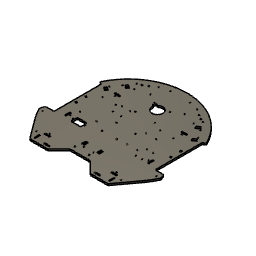
move_base_main_plate (Autodesk Fusion 360 design; units mm, degrees)
Autodesk Fusion 360 part; units mm, degrees
note: some values were not read from the file. Set by a fixed rule: which sketch regions a step uses.
sketch "スケッチ1" plane through (0, 0, 0) normal (0, 1, 0) x (1, 0, 0)
  circle A0 centre (0, 0) radius 220
  dimension "d1" = 440
  constraint coincident A0.centre origin
  measures "d1" diameter of A0
sketch "スケッチ2" plane through (0, 0, 0) normal (0, 1, 0) x (1, 0, 0)
  line L0 (-153.355, -39.3161) -> (-63.355, -39.3161)
  line L1 (-63.355, -39.3161) -> (-63.355, -141.3161)
  line L2 (-63.355, -141.3161) -> (-153.355, -141.3161)
  line L3 (-153.355, -141.3161) -> (-153.355, -39.3161)
  circle A0 centre (0, -150) radius 60.5
  line L4 (-174.2878, 56.0852) -> (-203.2878, 56.0852)
  line L5 (-203.2878, 56.0852) -> (-203.2878, -43.9148)
  line L6 (-203.2878, -43.9148) -> (-174.2878, -43.9148)
  line L7 (-174.2878, -43.9148) -> (-174.2878, 56.0852)
  line L8 (-147.9328, 18.2444) -> (-59.029, 18.2444)
  line L9 (-59.029, 18.2444) -> (-59.029, -18.7556)
  line L10 (-59.029, -18.7556) -> (-147.9328, -18.7556)
  line L11 (-147.9328, -18.7556) -> (-147.9328, 18.2444)
  dimension "d2" = 102
  dimension "d3" = 90
  dimension "d4" = 121
  dimension "d5" = 100
  dimension "d6" = 29
  dimension "d7" = 37
  dimension "d8" = 150
  constraint horizontal L0
  constraint vertical L1
  constraint horizontal L2
  constraint vertical L3
  constraint horizontal L4
  constraint vertical L5
  constraint horizontal L6
  constraint vertical L7
  constraint horizontal L8
  constraint vertical L9
  constraint horizontal L10
  constraint vertical L11
  measures "d2" distance of L0.start L2.end
  measures "d3" distance of L0.start L0.end
  measures "d4" diameter of A0
  measures "d5" distance of L4.end L5.end
  measures "d6" distance of L4.start L4.end
  measures "d7" distance of L8.end L9.end
  measures "d8" distance of A0.centre origin
sketch "スケッチ3" plane through (0, 0, 0) normal (0, 1, 0) x (1, 0, 0)
  line L0 (-159, 75) -> (-159, -75)
  line L1 (-159, -75) -> (-196.1505, -75)
  line L2 (-159, 75) -> (-168.0208, 75)
  line L3 (168.0208, 75) -> (159, 75)
  line L4 (159, 75) -> (159, -75)
  line L5 (159, -75) -> (196.1505, -75)
  arc A0 (168.0208, 75) -> (-168.0208, 75) centre (0, 0) ccw
  arc A1 (-196.1505, -75) -> (196.1505, -75) centre (0, 0) ccw
  circle A2 centre (0, -230) radius 75
  circle A3 centre (0, -210) radius 85
  line L6 (168.7454, -125) -> (68.3017, -260.5952)
  line L7 (-168.7454, -125) -> (-68.3017, -260.5952)
  line L8 (-122.8182, -187) -> (122.8182, -187)
  line L9 (-67, -187) -> (-32, -152)
  line L10 (-32, -152) -> (32, -152)
  line L11 (32, -152) -> (67, -187)
  point P0 (-159, 0)
  point P1 (159, 0)
  point P2 (0, -152)
  dimension "d9" = 150
  dimension "d10" = 159
  dimension "d12" = 159
  dimension "d13" = 184
  dimension "d14" = 210
  dimension "d64" = 150
  dimension "d65" = 230
  dimension "d66" = 210
  dimension "d67" = 170
  dimension "d109" = 187
  dimension "d164" = 64
  dimension "d165" = 35
  dimension "d166" = 135
  dimension "d167" = 135
  constraint vertical L0
  constraint perpendicular L0 L1
  constraint perpendicular L0 L2
  constraint horizontal L3
  constraint perpendicular L3 L4
  constraint perpendicular L4 L5
  constraint midpoint L0 P0
  constraint midpoint L4 P1
  constraint horizontal P1 A0.centre
  constraint horizontal P0 A0.centre
  constraint equal L0 L4
  constraint coincident A0.centre A1.centre
  constraint coincident L3.start A0.start
  constraint coincident L1.end A1.start
  constraint vertical A0.centre A2.centre
  constraint vertical A0.centre A3.centre
  constraint coincident A1 L7.start
  constraint coincident A3 L7.end
  constraint coincident A3 L6.end
  constraint coincident A1 L6.start
  constraint tangent A1 L6
  constraint tangent A3 L6
  constraint tangent A1 L7
  constraint tangent A3 L7
  constraint horizontal L8
  constraint coincident L6 L8.end
  constraint coincident L7 L8.start
  constraint coincident L8 L9.start
  constraint parallel L8 L10
  constraint coincident L8 L11.end
  constraint midpoint L10 P2
  constraint vertical A0.centre P2
  measures "d9" distance of L0.start L0.end
  measures "d10" distance of P0 A0.centre
  measures "d12" distance of P1 A0.centre
  measures "d13" radius of A0
  measures "d14" radius of A1
  measures "d64" diameter of A2
  measures "d65" distance of A0.centre A2.centre
  measures "d66" distance of A0.centre A3.centre
  measures "d67" diameter of A3
  measures "d109" distance of A0.centre L8
  measures "d164" distance of L9.end L10.end
  measures "d165" distance of L8 L10
  measures "d166" angle of L10 L11
  measures "d167" angle of L9 L10
extrude "押し出し1" add sketch "スケッチ3" along normal blind 5 contours L0 L1 L2 L3 L4 L5 A0 A1 A3 L8 | A1 L7 L8 | A3 L8 L9 L10 L11 | A1 L6 L8
sketch "スケッチ8" plane through (0, 5, 0) normal (0, 1, 0) x (-1, 0, 0)
  line L0 (-122.8182, 187) -> (-168.7454, 125)
  arc A0 (-168.7454, 125) -> (-196.1505, 75) centre (0, 0) ccw
  line L1 (-196.1505, 75) -> (-159, 75)
  line L2 (-159, 75) -> (-159, -75)
  arc A1 (-168.0208, -75) -> (168.0208, -75) centre (0, 0) ccw
  line L3 (159, -75) -> (159, 75)
  line L4 (159, 75) -> (196.1505, 75)
  line L5 (168.7454, 125) -> (122.8182, 187)
  line L6 (122.8182, 187) -> (67, 187)
  line L7 (31, -163) -> (-31, -163)
  line L8 (25, -106) -> (-25, -106)
  line L9 (-159, -75) -> (-168.0208, -75)
  line L10 (168.0208, -75) -> (159, -75)
  circle A2 centre (0, 0) radius 165
  line L11 (104.1506, -130.3942) -> (60.8494, -155.3942)
  line L12 (60.8494, -155.3942) -> (49.8494, -136.3416)
  line L13 (49.8494, -136.3416) -> (93.1506, -111.3416)
  line L14 (93.1506, -111.3416) -> (104.1506, -130.3942)
  line L15 (-60.8494, -155.3942) -> (-104.1506, -130.3942)
  line L16 (-104.1506, -130.3942) -> (-93.1507, -111.3416)
  line L17 (-93.1507, -111.3416) -> (-49.8494, -136.3416)
  line L18 (-49.8494, -136.3416) -> (-60.8494, -155.3942)
  line L19 (82.5, -142.8942) -> (0, 0)
  line L20 (0, 0) -> (-82.5, -142.8942)
  line L21 (0, 0) -> (0, -165)
  circle A3 centre (0, -91) radius 17.5
  line L22 (17.0919, -94.7574) -> (12.2438, -103.5036)
  line L23 (12.2438, -103.5036) -> (18.3661, -106.8973)
  line L24 (18.3661, -106.8973) -> (23.2142, -98.1511)
  line L25 (23.2142, -98.1511) -> (17.0919, -94.7574)
  line L26 (0, -91) -> (14.6678, -99.1305)
  line L27 (31, 138) -> (-15, 138)
  line L28 (-15, 138) -> (-15, 52)
  line L29 (-15, 52) -> (31, 52)
  line L30 (31, 52) -> (31, 138)
  line L31 (-30, -52) -> (30, -52)
  line L32 (30, -52) -> (30, 8)
  line L33 (30, 8) -> (-30, 8)
  line L34 (-30, 8) -> (-30, -52)
  line L35 (-30, -52) -> (30, 8) construction
  line L36 (30, -52) -> (-30, 8) construction
  line L37 (-60, -40) -> (-102, -40)
  line L38 (122, -40) -> (80, -40)
  line L39 (-45, -10) -> (-77, -10)
  line L40 (-77, -10) -> (-77, 49.5)
  line L41 (-77, 49.5) -> (-45, 49.5)
  line L42 (-45, 49.5) -> (-45, -10)
  line L43 (92.7583, -134.6621) -> (78.9019, -142.6621)
  line L44 (-78.9019, -142.6621) -> (-92.7583, -134.6621)
  arc A4 (-102.846, 122.5671) -> (102.846, 122.5671) centre (0, 0) ccw
  line L45 (0, 0) -> (102.846, 122.5671)
  line L46 (0, 0) -> (-102.846, 122.5671)
  line L47 (0, 0) -> (131.0643, -91.7722)
  line L48 (139.668, -79.4849) -> (122.4607, -104.0595)
  line L49 (0, 0) -> (-131.0643, -91.7722)
  line L50 (-122.4607, -104.0595) -> (-139.668, -79.4849)
  line L51 (114.185, -114.1349) -> (104.3552, -107.252)
  line L52 (104.3552, -107.252) -> (108.9438, -100.6988)
  line L53 (108.9438, -100.6988) -> (118.7736, -107.5817)
  line L54 (118.7736, -107.5817) -> (114.185, -114.1349)
  line L55 (146.3053, -68.2624) -> (136.4755, -61.3795)
  line L56 (136.4755, -61.3795) -> (131.8869, -67.9327)
  line L57 (131.8869, -67.9327) -> (141.7167, -74.8156)
  line L58 (141.7167, -74.8156) -> (146.3053, -68.2624)
  line L59 (141.7167, -74.8156) -> (118.7736, -107.5817)
  line L60 (-118.7736, -107.5817) -> (-141.7167, -74.8156)
  line L61 (-118.7736, -107.5817) -> (-114.185, -114.1349)
  line L62 (-114.185, -114.1349) -> (-104.3552, -107.252)
  line L63 (-104.3552, -107.252) -> (-108.9438, -100.6988)
  line L64 (-108.9438, -100.6988) -> (-118.7736, -107.5817)
  line L65 (-141.7167, -74.8156) -> (-146.3053, -68.2624)
  line L66 (-146.3053, -68.2624) -> (-136.4755, -61.3795)
  line L67 (-136.4755, -61.3795) -> (-131.8869, -67.9327)
  line L68 (-131.8869, -67.9327) -> (-141.7167, -74.8156)
  line L69 (-90, 32) -> (-110, 32)
  line L70 (-110, 32) -> (-110, 67)
  line L71 (-110, 67) -> (-90, 67)
  line L72 (-90, 67) -> (-90, 32)
  arc A5 (196.1505, 75) -> (168.7454, 125) centre (0, 0) ccw
  line L73 (66, -45.5) -> (40, -45.5)
  line L74 (40, -45.5) -> (40, -17)
  line L75 (40, -17) -> (66, -17)
  line L76 (66, -17) -> (66, -45.5)
  line L77 (67, 187) -> (32, 152)
  line L78 (32, 152) -> (-32, 152)
  line L79 (-32, 152) -> (-67, 187)
  line L80 (-67, 187) -> (-122.8182, 187)
  line L81 (49.8494, -136.3416) -> (58.5096, -131.3416)
  line L82 (58.5096, -131.3416) -> (53.5096, -122.6814)
  line L83 (53.5096, -122.6814) -> (44.8494, -127.6814)
  line L84 (44.8494, -127.6814) -> (49.8494, -136.3416)
  line L85 (-49.8494, -136.3416) -> (-58.5096, -131.3416)
  line L86 (-58.5096, -131.3416) -> (-53.5096, -122.6814)
  line L87 (-53.5096, -122.6814) -> (-44.8494, -127.6814)
  line L88 (-44.8494, -127.6814) -> (-49.8494, -136.3416)
  line L89 (15, 125) -> (-15, 125)
  line L90 (20, 119) -> (-20, 119)
  line L91 (20, 119) -> (28, 119)
  line L92 (28, 119) -> (28, 107)
  line L93 (28, 107) -> (20, 107)
  line L94 (20, 107) -> (20, 119)
  line L95 (-20, 119) -> (-28, 119)
  line L96 (-28, 119) -> (-28, 107)
  line L97 (-28, 107) -> (-20, 107)
  line L98 (-20, 107) -> (-20, 119)
  circle A6 centre (87, 177) radius 1.6
  circle A7 centre (72, 177) radius 1.6
  line L99 (87, 178.6) -> (72, 178.6)
  line L100 (72, 178.6) -> (72, 175.4)
  line L101 (72, 175.4) -> (87, 175.4)
  line L102 (87, 175.4) -> (87, 178.6)
  line L103 (115.4, 177) -> (118.6, 177)
  line L104 (118.6, 177) -> (118.6, 162)
  line L105 (118.6, 162) -> (115.4, 162)
  line L106 (115.4, 162) -> (115.4, 177)
  circle A8 centre (117, 177) radius 1.6
  circle A9 centre (117, 162) radius 1.6
  circle A10 centre (-72, 177) radius 1.6
  circle A11 centre (-87, 177) radius 1.6
  circle A12 centre (-117, 177) radius 1.6
  circle A13 centre (-117, 162) radius 1.6
  line L107 (-72, 175.4) -> (-87, 175.4)
  line L108 (-87, 175.4) -> (-87, 178.6)
  line L109 (-87, 178.6) -> (-72, 178.6)
  line L110 (-72, 178.6) -> (-72, 175.4)
  line L111 (-115.4, 177) -> (-118.6, 177)
  line L112 (-118.6, 177) -> (-118.6, 162)
  line L113 (-118.6, 162) -> (-115.4, 162)
  line L114 (-115.4, 162) -> (-115.4, 177)
  line L115 (75, 75) -> (106, 75)
  line L116 (106, 75) -> (106, 55)
  line L117 (106, 55) -> (75, 55)
  line L118 (75, 55) -> (75, 75)
  line L119 (75, 75) -> (106, 55) construction
  line L120 (106, 75) -> (75, 55) construction
  line L121 (109, 65) -> (72, 65)
  line L122 (117, 35) -> (65, 35)
  point P0 (0, -163)
  point P1 (0, -106)
  point P2 (0, -165)
  point P3 (82.5, -142.8942)
  point P4 (-82.5, -142.8942)
  point P5 (8, 52)
  point P6 (0, -22)
  point P7 (0, -160)
  point P8 (102.846, 122.5671)
  point P9 (-102.846, 122.5671)
  point P10 (131.0643, -91.7722)
  point P11 (-131.0643, -91.7722)
  point P12 (0, -157)
  point P13 (130.2452, -91.1987)
  point P14 (-130.2452, -91.1987)
  point P15 (98.9893, 117.9708)
  point P16 (-98.9893, 117.9708)
  point P17 (0, 125)
  point P18 (0, 119)
  point P19 (90.5, 65)
  dimension "d68" = 163
  dimension "d69" = 62
  dimension "d70" = 50
  dimension "d71" = 57
  dimension "d75" = 330
  dimension "d78" = 30
  dimension "d79" = 30
  dimension "d80" = 50
  dimension "d81" = 35
  dimension "d82" = 15
  dimension "d83" = 7
  dimension "d84" = 10
  dimension "d85" = 61
  dimension "d101" = 22
  dimension "d102" = 86
  dimension "d103" = 46
  dimension "d104" = 52
  dimension "d105" = 8
  dimension "d110" = 60
  dimension "d111" = 22
  dimension "d112" = 42
  dimension "d113" = 60
  dimension "d114" = 80
  dimension "d115" = 40
  dimension "d116" = 32
  dimension "d117" = 59.5
  dimension "d118" = 45
  dimension "d119" = 10
  dimension "d120" = 2
  dimension "d121" = 13
  dimension "d122" = 3
  dimension "d123" = 3
  dimension "d124" = 13
  dimension "d125" = 2
  dimension "d129" = 160
  dimension "d130" = 55
  dimension "d131" = 85
  dimension "d132" = 55
  dimension "d133" = 85
  dimension "d141" = 1
  dimension "d142" = 1
  dimension "d145" = 20
  dimension "d146" = 35
  dimension "d157" = 26
  dimension "d158" = 28.5
  dimension "d159" = 40
  dimension "d160" = 17
  dimension "d175" = 10
  dimension "d176" = 12
  dimension "d178" = 20
  dimension "d179" = 125
  dimension "d180" = 40
  dimension "d181" = 30
  dimension "d182" = 6
  dimension "d183" = 12
  dimension "d184" = 8
  dimension "d185" = 3.2
  dimension "d186" = 3.2
  dimension "d187" = 10
  dimension "d188" = 15
  dimension "d189" = 5
  dimension "d190" = 10
  dimension "d191" = 50
  dimension "d192" = 15
  dimension "d193" = 3.2
  dimension "d194" = 3.2
  dimension "d195" = 5
  dimension "d196" = 10
  dimension "d197" = 15
  dimension "d198" = 50
  dimension "d199" = 10
  dimension "d200" = 15
  dimension "d201" = 31
  dimension "d202" = 20
  dimension "d203" = 37
  dimension "d204" = 75
  dimension "d205" = 65
  dimension "d219" = 8
  dimension "d223" = 90
  dimension "d224" = 32
  dimension "d225" = 52
  dimension "d226" = 65
  dimension "d227" = 35
  constraint horizontal L7
  constraint horizontal L8
  constraint midpoint L7 P0
  constraint midpoint L8 P1
  constraint vertical A0.centre P1
  constraint vertical A0.centre P0
  constraint concentric A0 A2
  constraint coincident A2 P2
  constraint perpendicular L11 L12
  constraint parallel L11 L13
  constraint parallel L12 L14
  constraint perpendicular L15 L16
  constraint parallel L15 L17
  constraint parallel L16 L18
  constraint coincident A2 P3
  constraint coincident A0.centre A1.centre
  constraint coincident A2 P4
  constraint coincident P2 L21.end
  constraint midpoint L11 P3
  constraint midpoint L15 P4
  constraint coincident P4 L20.end
  constraint coincident P3 L19.start
  constraint tangent A2 L11
  constraint tangent A2 L15
  constraint equal L13 L17
  constraint perpendicular L22 L23
  constraint parallel L22 L24
  constraint parallel L23 L25
  constraint coincident A3 L22.end
  constraint coincident A3 L22.start
  constraint vertical P1 A3.centre
  constraint coincident A3.centre L26.start
  constraint perpendicular L22 L26
  constraint coincident L22 L26.end
  constraint vertical L21
  constraint equal L12 L18
  constraint horizontal L27
  constraint vertical L28
  constraint horizontal L29
  constraint midpoint L29 P5
  constraint horizontal L31
  constraint perpendicular L31 L32
  constraint parallel L31 L33
  constraint parallel L32 L34
  constraint coincident L35 P6
  constraint coincident L36 P6
  constraint vertical A0.centre P6
  constraint equal L31 L32
  constraint horizontal L37
  constraint horizontal L38
  constraint equal L37 L38
  constraint collinear L37 L38
  constraint horizontal L39
  constraint vertical L40
  constraint horizontal L41
  constraint vertical L42
  constraint parallel L11 L43
  constraint perpendicular L20 L44
  constraint coincident L21 P7
  constraint coincident P7 A4
  constraint coincident P9 A4.start
  constraint coincident P8 A4.end
  constraint coincident A4 P10
  constraint perpendicular L47 L48
  constraint midpoint L48 P10
  constraint coincident P10 L47.end
  constraint coincident A4 P11
  constraint midpoint L50 P11
  constraint coincident P11 L49.end
  constraint perpendicular L49 L50
  constraint coincident L21 P12
  constraint perpendicular L51 L52
  constraint parallel L51 L53
  constraint parallel L52 L54
  constraint perpendicular L55 L56
  constraint parallel L55 L57
  constraint parallel L56 L58
  constraint coincident L47 P13
  constraint equal L52 L56
  constraint equal L53 L57
  constraint perpendicular L53 L59
  constraint midpoint P13 L59
  constraint perpendicular L47 L59
  constraint perpendicular L57 L59
  constraint midpoint L60 P14
  constraint coincident L49 P14
  constraint perpendicular L49 L60
  constraint perpendicular L61 L62
  constraint parallel L61 L63
  constraint parallel L62 L64
  constraint parallel L60 L61
  constraint perpendicular L65 L66
  constraint parallel L65 L67
  constraint parallel L66 L68
  constraint perpendicular L49 L65
  constraint equal L62 L66
  constraint equal L63 L67
  constraint coincident L46 P16
  constraint coincident L45 P15
  constraint horizontal L69
  constraint vertical L70
  constraint horizontal L71
  constraint vertical L72
  constraint horizontal L73
  constraint vertical L74
  constraint horizontal L75
  constraint vertical L76
  constraint perpendicular L81 L82
  constraint parallel L81 L83
  constraint parallel L82 L84
  constraint coincident L13 L81.end
  constraint perpendicular L85 L86
  constraint parallel L85 L87
  constraint parallel L86 L88
  constraint coincident L17 L85.end
  constraint equal L83 L84
  constraint equal L87 L88
  constraint equal L84 L88
  constraint equal L51 L62
  constraint equal L52 L63
  constraint equal L59 L60
  constraint horizontal L89
  constraint midpoint L89 P17
  constraint vertical A0.centre P17
  constraint horizontal L90
  constraint midpoint L90 P18
  constraint vertical P17 P18
  constraint horizontal L91
  constraint vertical L92
  constraint horizontal L93
  constraint vertical L94
  constraint horizontal L95
  constraint vertical L96
  constraint horizontal L97
  constraint vertical L98
  constraint collinear L93 L97
  constraint equal L93 L97
  constraint horizontal L99
  constraint vertical L100
  constraint horizontal L101
  constraint vertical L102
  constraint horizontal L103
  constraint vertical L104
  constraint horizontal L105
  constraint vertical L106
  constraint tangent A6 L101
  constraint tangent A6 L99
  constraint tangent A7 L99
  constraint tangent A7 L101
  constraint midpoint A6.centre L102
  constraint midpoint A7.centre L100
  constraint tangent L106 A9
  constraint tangent L104 A9
  constraint tangent L104 A8
  constraint tangent L106 A8
  constraint midpoint L105 A9.centre
  constraint midpoint L103 A8.centre
  constraint horizontal L107
  constraint vertical L108
  constraint horizontal L109
  constraint vertical L110
  constraint horizontal L111
  constraint vertical L112
  constraint horizontal L113
  constraint vertical L114
  constraint tangent A10 L107
  constraint tangent A11 L107
  constraint tangent A11 L109
  constraint tangent A10 L109
  constraint tangent A12 L114
  constraint tangent A12 L112
  constraint tangent A13 L112
  constraint tangent A13 L114
  constraint midpoint A13.centre L113
  constraint midpoint A12.centre L111
  constraint midpoint A11.centre L108
  constraint midpoint A10.centre L110
  constraint horizontal L115
  constraint perpendicular L115 L116
  constraint parallel L115 L117
  constraint parallel L116 L118
  constraint coincident L119 P19
  constraint coincident L120 P19
  constraint horizontal L121
  constraint midpoint P19 L121
  constraint vertical L30
  constraint horizontal L122
  measures "d68" distance of A0.centre P0
  measures "d69" distance of L7.start L7.end
  measures "d70" distance of L8.start L8.end
  measures "d71" distance of L7 L8
  measures "d75" diameter of A2
  measures "d78" angle of L19 L21
  measures "d79" angle of L20 L21
  measures "d80" distance of L12.end L13.end
  measures "d81" diameter of A3
  measures "d82" distance of L8 A3.centre
  measures "d83" distance of L22.start L24.end
  measures "d84" distance of L23.end L24.end
  measures "d85" angle of L21 L26
  measures "d101" distance of L11.start L13.end
  measures "d102" distance of L27.end L28.end
  measures "d103" distance of L28.end L29.end
  measures "d104" distance of A0.centre L29
  measures "d105" horizontal distance of A0.centre P5
  measures "d110" distance of L31.end L32.end
  measures "d111" distance of A0.centre P6
  measures "d112" distance of L37.start L37.end
  measures "d113" horizontal distance of A0.centre L37.start
  measures "d114" horizontal distance of A0.centre L38.end
  measures "d115" distance of A0.centre L37
  measures "d116" distance of L39.start L39.end
  measures "d117" distance of L39.end L40.end
  measures "d118" distance of A0.centre L42
  measures "d119" distance of A0.centre L39
  measures "d120" distance of L11 L43
  measures "d121" distance of L19 L43.start
  measures "d122" distance of L19 L43.end
  measures "d123" distance of L20 L44.start
  measures "d124" distance of L20 L44.end
  measures "d125" distance of L15 L44
  measures "d129" radius of A4
  measures "d130" angle of L21 L47
  measures "d131" angle of L45 L47
  measures "d132" angle of L21 L49
  measures "d133" angle of L46 L49
  measures "d141" distance of L48 L59
  measures "d142" distance of L50 L60
  measures "d145" distance of L69.start L69.end
  measures "d146" distance of L69.start L71.end
  measures "d157" distance of L73.start L73.end
  measures "d158" distance of L73.start L75.end
  measures "d159" distance of A0.centre L74
  measures "d160" distance of A0.centre L75
  measures "d175" distance of L12.end L83.end
  measures "d176" distance of L55.start L55.end
  measures "d178" distance of L47 L57
  measures "d179" distance of A0.centre L89
  measures "d180" distance of L90.start L90.end
  measures "d181" distance of L89.start L89.end
  measures "d182" distance of L89 L90
  measures "d183" distance of L91.end L92.end
  measures "d184" distance of L92.end L93.end
  measures "d185" diameter of A6
  measures "d186" diameter of A8
  measures "d187" distance of L6 A6.centre
  measures "d188" distance of A6.centre A7.centre
  measures "d189" horizontal distance of L6.end A7.centre
  measures "d190" vertical distance of L6.end A8.centre
  measures "d191" horizontal distance of L6.end A8.centre
  measures "d192" distance of A8.centre A9.centre
  measures "d193" diameter of A10
  measures "d194" diameter of A13
  measures "d195" horizontal distance of L79.end A10.centre
  measures "d196" vertical distance of L79.end A10.centre
  measures "d197" distance of A10.centre A11.centre
  measures "d198" horizontal distance of L79.end A12.centre
  measures "d199" vertical distance of L79.end A12.centre
  measures "d200" distance of A12.centre A13.centre
  measures "d201" distance of L116.end L117.end
  measures "d202" distance of L115.end L116.end
  measures "d203" distance of L121.start L121.end
  measures "d204" distance of A0.centre L118
  measures "d205" distance of A0.centre L121
  measures "d219" distance of L62.end L63.end
  measures "d223" distance of A0.centre L72
  measures "d224" distance of A0.centre L69
  measures "d225" distance of L122.start L122.end
  measures "d226" horizontal distance of A0.centre L122.end
  measures "d227" distance of A0.centre L122
hole "穴5" at (25, 5, -106) at (-25, 5, -106) at (-31, 5, -163) at (31, 5, -163) at (-104.1506, 5, -130.3942) at (-93.1506, 5, -111.3416) at (-60.8494, 5, -155.3942) at (60.8494, 5, -155.3942) at (104.1506, 5, -130.3942) at (93.1507, 5, -111.3416) at (60, 5, -40) at (102, 5, -40) at (-80, 5, -40) at (-122, 5, -40) at (45, 5, -10) at (77, 5, -10) at (77, 5, 49.5) at (45, 5, 49.5) at (-122.4607, 5, -104.0595) at (-139.668, 5, -79.4849) at (122.4607, 5, -104.0595) at (139.668, 5, -79.4849) at (90, 5, 32) at (110, 5, 32) at (110, 5, 67) at (90, 5, 67) at (-30, 5, -52) at (-30, 5, 8) at (30, 5, 8) at (30, 5, -52) at (-66, 5, -45.5) at (-40, 5, -45.5) at (-40, 5, -17) at (-66, 5, -17) at (-53.5096, 5, -122.6814) at (53.5096, 5, -122.6814) at (-15, 5, 125) at (15, 5, 125) direction (0, -1, 0) diameter 3.2 end through all
extrude "押し出し2" cut sketch "スケッチ8" against normal through all contours A4 L66 L67 L68 | A4 L65 L66 L68 | A4 L55 L57 L58 | A4 L55 L56 L57 | A4 L61 L62 L64 | A4 L62 L63 L64 | A4 L51 L52 L53 | A4 L51 L53 L54 | L21 A3 L22 L26 | L8 L21 A3 | L8 L21 A3 L22 L26 | L8 L21 A3 | L8 L21 A3 | A3 L22 | L8 A3 L23 L24 L25 | L8 L23 L24 | L91 L92 L93 L94 | L95 L96 L97 L98 | A6 L102 | A6 L102 | A6 A7 L99 L101 | A7 L100 | A7 L100 | L103 A8 | L104 L106 A8 A9 | L103 A8 | L105 A9 | L105 A9 | A10 L110 | A10 L110 | A10 A11 L107 L109 | A11 L108 | A11 L108 | A12 L111 | A12 A13 L112 L114 | A12 L111 | A13 L113 | A13 L113 | L115 L116 L118 L121 | L116 L117 L118 L121
sketch "スケッチ9" plane through (0, 5, 0) normal (0, 1, 0) x (-1, 0, 0)
  line L0 (23.2142, -98.1511) -> (18.3661, -106.8973)
  line L1 (18.3661, -106.8973) -> (12.2438, -103.5036)
  arc A0 (17.0919, -94.7574) -> (12.2438, -103.5036) centre (0, -91) ccw
  line L2 (17.0919, -94.7574) -> (23.2142, -98.1511)
  circle A1 centre (-104.1506, -130.3942) radius 1.6
  circle A2 centre (104.1506, -130.3942) radius 1.6
  circle A3 centre (31, -163) radius 1.6
  circle A4 centre (-25, -106) radius 1.6
  circle A5 centre (25, -106) radius 1.6
  circle A6 centre (-31, -163) radius 1.6
  circle A7 centre (93.1506, -111.3416) radius 1.6
  circle A8 centre (60.8494, -155.3942) radius 1.6
  circle A9 centre (-60.8494, -155.3942) radius 1.6
  circle A10 centre (-93.1507, -111.3416) radius 1.6
  line L3 (-122.8182, 187) -> (-168.7454, 125)
  arc A11 (-168.7454, 125) -> (-196.1505, 75) centre (0, 0) ccw
  line L4 (-196.1505, 75) -> (-159, 75)
  line L5 (-159, 75) -> (-159, -75)
  line L6 (-159, -75) -> (-168.0208, -75)
  arc A12 (-168.0208, -75) -> (168.0208, -75) centre (0, 0) ccw
  line L7 (168.0208, -75) -> (159, -75)
  line L8 (159, -75) -> (159, 75)
  line L9 (159, 75) -> (196.1505, 75)
  line L10 (168.7454, 125) -> (122.8182, 187)
  line L11 (122.8182, 187) -> (67, 187)
  line L12 (-130, -70) -> (130, -70)
  line L13 (130, -70) -> (130, 150)
  line L14 (130, 150) -> (-130, 150)
  line L15 (-130, 150) -> (-130, -70)
  line L16 (-130, -70) -> (130, 150) construction
  line L17 (130, -70) -> (-130, 150) construction
  line L18 (123, 60) -> (123, -63)
  line L19 (123, -63) -> (-123, -63)
  line L20 (-123, -63) -> (-123, 60)
  circle A13 centre (80, -40) radius 1.6
  circle A14 centre (-60, -40) radius 1.6
  circle A15 centre (-102, -40) radius 1.6
  circle A16 centre (122, -40) radius 1.6
  circle A17 centre (-77, 49.5) radius 1.6
  circle A18 centre (-45, -10) radius 1.6
  circle A19 centre (-77, -10) radius 1.6
  circle A20 centre (-45, 49.5) radius 1.6
  circle A21 centre (-122.4607, -104.0595) radius 1.6
  circle A22 centre (122.4607, -104.0595) radius 1.6
  circle A23 centre (139.668, -79.4849) radius 1.6
  circle A24 centre (-139.668, -79.4849) radius 1.6
  line L21 (-108.9438, -100.6988) -> (-104.3552, -107.252)
  line L22 (-104.3552, -107.252) -> (-114.185, -114.1349)
  line L23 (-114.185, -114.1349) -> (-118.7736, -107.5817)
  line L24 (-118.7736, -107.5817) -> (-108.9438, -100.6988)
  line L25 (141.7167, -74.8156) -> (131.8869, -67.9327)
  line L26 (131.8869, -67.9327) -> (136.4755, -61.3795)
  line L27 (136.4755, -61.3795) -> (146.3053, -68.2624)
  line L28 (146.3053, -68.2624) -> (141.7167, -74.8156)
  line L29 (118.7736, -107.5817) -> (114.185, -114.1349)
  line L30 (114.185, -114.1349) -> (104.3552, -107.252)
  line L31 (104.3552, -107.252) -> (108.9438, -100.6988)
  line L32 (108.9438, -100.6988) -> (118.7736, -107.5817)
  line L33 (-131.8869, -67.9327) -> (-141.7167, -74.8156)
  line L34 (-141.7167, -74.8156) -> (-146.3053, -68.2624)
  line L35 (-146.3053, -68.2624) -> (-136.4755, -61.3795)
  line L36 (-136.4755, -61.3795) -> (-131.8869, -67.9327)
  circle A25 centre (-110, 67) radius 1.6
  circle A26 centre (-90, 32) radius 1.6
  circle A27 centre (-110, 32) radius 1.6
  circle A28 centre (-90, 67) radius 1.6
  arc A29 (196.1505, 75) -> (168.7454, 125) centre (0, 0) ccw
  circle A30 centre (-30, 8) radius 1.6
  circle A31 centre (30, -52) radius 1.6
  circle A32 centre (30, 8) radius 1.6
  circle A33 centre (-30, -52) radius 1.6
  line L37 (105, 142.5) -> (-105, 142.5)
  circle A34 centre (40, -17) radius 1.6
  circle A35 centre (66, -45.5) radius 1.6
  circle A36 centre (40, -45.5) radius 1.6
  circle A37 centre (66, -17) radius 1.6
  line L38 (97, -72) -> (113, -72)
  line L39 (113, -72) -> (113, -68)
  line L40 (113, -68) -> (97, -68)
  line L41 (97, -68) -> (97, -72)
  line L42 (97, -72) -> (113, -68) construction
  line L43 (113, -72) -> (97, -68) construction
  line L44 (-113, -72) -> (-97, -72)
  line L45 (-97, -72) -> (-97, -68)
  line L46 (-97, -68) -> (-113, -68)
  line L47 (-113, -68) -> (-113, -72)
  line L48 (-113, -72) -> (-97, -68) construction
  line L49 (-97, -72) -> (-113, -68) construction
  line L50 (97, 148) -> (113, 148)
  line L51 (113, 148) -> (113, 152)
  line L52 (113, 152) -> (97, 152)
  line L53 (97, 152) -> (97, 148)
  line L54 (97, 148) -> (113, 152) construction
  line L55 (113, 148) -> (97, 152) construction
  line L56 (-113, 148) -> (-97, 148)
  line L57 (-97, 148) -> (-97, 152)
  line L58 (-97, 152) -> (-113, 152)
  line L59 (-113, 152) -> (-113, 148)
  line L60 (-113, 148) -> (-97, 152) construction
  line L61 (-97, 148) -> (-113, 152) construction
  line L62 (-132, 52) -> (-128, 52)
  line L63 (-128, 52) -> (-128, 68)
  line L64 (-128, 68) -> (-132, 68)
  line L65 (-132, 68) -> (-132, 52)
  line L66 (-132, 52) -> (-128, 68) construction
  line L67 (-128, 52) -> (-132, 68) construction
  line L68 (128, 52) -> (132, 52)
  line L69 (132, 52) -> (132, 68)
  line L70 (132, 68) -> (128, 68)
  line L71 (128, 68) -> (128, 52)
  line L72 (128, 52) -> (132, 68) construction
  line L73 (132, 52) -> (128, 68) construction
  line L74 (67, 187) -> (32, 152)
  line L75 (32, 152) -> (-32, 152)
  line L76 (-32, 152) -> (-67, 187)
  line L77 (-67, 187) -> (-122.8182, 187)
  circle A38 centre (53.5096, -122.6814) radius 1.6
  circle A39 centre (-53.5096, -122.6814) radius 1.6
  circle A40 centre (15, 125) radius 1.6
  circle A41 centre (-15, 125) radius 1.6
  line L78 (20, 107) -> (20, 119)
  line L79 (20, 119) -> (28, 119)
  line L80 (28, 119) -> (28, 107)
  line L81 (28, 107) -> (20, 107)
  line L82 (-20, 107) -> (-28, 107)
  line L83 (-28, 107) -> (-28, 119)
  line L84 (-28, 119) -> (-20, 119)
  line L85 (-20, 119) -> (-20, 107)
  arc A42 (72, 178.6) -> (72, 175.4) centre (72, 177) ccw
  line L86 (72, 178.6) -> (87, 178.6)
  arc A43 (87, 175.4) -> (87, 178.6) centre (87, 177) ccw
  line L87 (87, 175.4) -> (72, 175.4)
  line L88 (118.6, 177) -> (118.6, 162)
  arc A44 (115.4, 162) -> (118.6, 162) centre (117, 162) ccw
  line L89 (115.4, 162) -> (115.4, 177)
  arc A45 (118.6, 177) -> (115.4, 177) centre (117, 177) ccw
  line L90 (-72, 175.4) -> (-87, 175.4)
  arc A46 (-87, 178.6) -> (-87, 175.4) centre (-87, 177) ccw
  line L91 (-87, 178.6) -> (-72, 178.6)
  arc A47 (-72, 175.4) -> (-72, 178.6) centre (-72, 177) ccw
  arc A48 (-118.6, 162) -> (-115.4, 162) centre (-117, 162) ccw
  line L92 (-118.6, 162) -> (-118.6, 177)
  arc A49 (-115.4, 177) -> (-118.6, 177) centre (-117, 177) ccw
  line L93 (-115.4, 177) -> (-115.4, 162)
  line L94 (75, 55) -> (75, 75)
  line L95 (75, 75) -> (106, 75)
  line L96 (106, 75) -> (106, 55)
  line L97 (106, 55) -> (75, 55)
  line L98 (149.05, -15.6) -> (130, -15.6)
  line L99 (130, -15.6) -> (130, 15.6)
  line L100 (130, 15.6) -> (149.05, 15.6)
  line L101 (149.05, 15.6) -> (149.05, -15.6)
  line L102 (-130, -15.6) -> (-149.05, -15.6)
  line L103 (-149.05, -15.6) -> (-149.05, 15.6)
  line L104 (-149.05, 15.6) -> (-130, 15.6)
  line L105 (-130, 15.6) -> (-130, -15.6)
  point P0 (0, 40)
  point P1 (105, -63)
  point P2 (-105, -63)
  point P3 (105, -70)
  point P4 (-105, -70)
  point P5 (105, 150)
  point P6 (-105, 150)
  point P7 (-130, 60)
  point P8 (130, 60)
  point P9 (130, 0)
  point P10 (-130, 0)
  dimension "d89" = 40
  dimension "d90" = 260
  dimension "d91" = 220
  dimension "d92" = 60
  dimension "d93" = 105
  dimension "d94" = 105
  dimension "d95" = 7
  dimension "d96" = 7
  dimension "d97" = 7
  dimension "d156" = 7.5
  dimension "d161" = 16
  dimension "d162" = 4
  dimension "d231" = 19.05
  dimension "d232" = 31.2
  constraint horizontal L12
  constraint perpendicular L12 L13
  constraint parallel L12 L14
  constraint parallel L13 L15
  constraint coincident L16 P0
  constraint coincident L17 P0
  constraint vertical A11.centre P0
  constraint vertical L18
  constraint perpendicular L18 L19
  constraint perpendicular L19 L20
  constraint coincident L19 P1
  constraint coincident L19 P2
  constraint horizontal L18.start L20.end
  constraint horizontal L37
  constraint vertical P1 L37.start
  constraint vertical P2 L37.end
  constraint horizontal L38
  constraint perpendicular L38 L39
  constraint parallel L38 L40
  constraint parallel L39 L41
  constraint coincident L42 P3
  constraint coincident L43 P3
  constraint coincident L12 P3
  constraint vertical P1 P3
  constraint horizontal L44
  constraint perpendicular L44 L45
  constraint parallel L44 L46
  constraint parallel L45 L47
  constraint coincident L48 P4
  constraint coincident L49 P4
  constraint coincident L12 P4
  constraint vertical P2 P4
  constraint horizontal L50
  constraint perpendicular L50 L51
  constraint parallel L50 L52
  constraint parallel L51 L53
  constraint coincident L54 P5
  constraint coincident L55 P5
  constraint coincident L14 P5
  constraint horizontal L56
  constraint perpendicular L56 L57
  constraint parallel L56 L58
  constraint parallel L57 L59
  constraint coincident L60 P6
  constraint coincident L61 P6
  constraint coincident L14 P6
  constraint horizontal L62
  constraint perpendicular L62 L63
  constraint parallel L62 L64
  constraint parallel L63 L65
  constraint coincident L66 P7
  constraint coincident L67 P7
  constraint coincident L15 P7
  constraint horizontal L68
  constraint perpendicular L68 L69
  constraint parallel L68 L70
  constraint parallel L69 L71
  constraint coincident L72 P8
  constraint coincident L73 P8
  constraint coincident L13 P8
  constraint horizontal L18.start P8
  constraint horizontal L20.end P7
  constraint vertical L37.end P6
  constraint vertical L37.start P5
  constraint equal L40 L46
  constraint equal L40 L71
  constraint equal L50 L71
  constraint equal L46 L63
  constraint equal L56 L63
  constraint equal L41 L45
  constraint equal L45 L62
  constraint equal L59 L62
  constraint equal L41 L68
  constraint equal L51 L68
  constraint horizontal L98
  constraint vertical L99
  constraint horizontal L100
  constraint vertical L101
  constraint midpoint L99 P9
  constraint horizontal A11.centre P9
  constraint coincident L13 P9
  constraint horizontal L102
  constraint vertical L103
  constraint horizontal L104
  constraint vertical L105
  constraint midpoint L105 P10
  constraint horizontal A11.centre P10
  constraint coincident L15 P10
  constraint equal L98 L102
  constraint equal L101 L103
  measures "d89" distance of A11.centre P0
  measures "d90" distance of L12.start L12.end
  measures "d91" distance of L12.start L14.end
  measures "d92" vertical distance of A11.centre L18.start
  measures "d93" horizontal distance of A11.centre P1
  measures "d94" horizontal distance of A11.centre P2
  measures "d95" distance of L12 L19
  measures "d96" distance of L15 L20
  measures "d97" distance of L13 L18
  measures "d156" distance of L14 L37
  measures "d161" distance of L38.start L38.end
  measures "d162" distance of L38.start L40.end
  measures "d231" distance of L98.start L98.end
  measures "d232" distance of L98.start L100.end
hole "穴6" at (-123, 5, 60) at (-105, 5, -63) at (105, 5, -63) at (123, 5, 60) at (-105, 5, 142.5) at (105, 5, 142.5) at (-109, 5, 65) at (-72, 5, 65) direction (0, -1, 0) diameter 3.2 end through all
hole "穴7" at (15, 5, 52) at (-31, 5, 52) at (-31, 5, 138) at (15, 5, 138) at (92.7583, 5, -134.6621) at (78.9019, 5, -142.6621) at (-92.7583, 5, -134.6621) at (-78.9019, 5, -142.6621) direction (0, -1, 0) diameter 4.3 end through all
chamfer "面取り1" distance 10 distance2 15 1 edges at (-196.1505, 2.5, 75) measured on face at (-171.3835, 1.6667, 75)
chamfer "面取り2" distance 15 distance2 10 1 edges at (196.1505, 2.5, 75) measured on face at (172.4502, 1.6667, 119.837)
fillet "フィレット1" radius 3 20 edges at (168.0208, 2.5, -75) (159, 2.5, -75) (159, 2.5, 75) (-159, 2.5, 75) (-159, 2.5, -75) (-168.0208, 2.5, -75) (-122.8182, 2.5, 187) (122.8182, 2.5, 187) (190.2963, 2.5, 88.8105) (186.1505, 2.5, 75) (-190.2963, 2.5, 88.8105) (-186.1505, 2.5, 75) (-67, 2.5, 187) (-32, 2.5, 152) (67, 2.5, 187) (32, 2.5, 152) (-75, 2.5, 55) (-106, 2.5, 55) (-106, 2.5, 75) (-75, 2.5, 75)
extrude "押し出し3" cut sketch "スケッチ9" against normal through all contours L12 L45 L46 L47 | L12 L44 L45 L47 | L12 L39 L40 L41 | L12 L38 L39 L41 | L15 L62 L64 L65 | L15 L62 L63 L64 | L14 L57 L58 L59 | L14 L56 L57 L59 | L13 L68 L70 L71 | L13 L68 L69 L70 | L14 L51 L52 L53 | L14 L50 L51 L53
sketch "スケッチ10" plane through (0, 0, 0) normal (0, -1, 0) x (1, 0, 0)
  line L0 (97, 152) -> (113, 152)
  line L1 (113, 152) -> (113, 148)
  line L2 (113, 148) -> (97, 148)
  line L3 (97, 148) -> (97, 152)
  line L4 (-113, -68) -> (-97, -68)
  line L5 (-97, -68) -> (-97, -72)
  line L6 (-97, -72) -> (-113, -72)
  line L7 (-113, -72) -> (-113, -68)
  line L8 (128, 68) -> (132, 68)
  line L9 (132, 68) -> (132, 52)
  line L10 (132, 52) -> (128, 52)
  line L11 (128, 52) -> (128, 68)
  line L12 (-113, 152) -> (-97, 152)
  line L13 (-97, 152) -> (-97, 148)
  line L14 (-97, 148) -> (-113, 148)
  line L15 (-113, 148) -> (-113, 152)
  line L16 (-132, 68) -> (-128, 68)
  line L17 (-128, 68) -> (-128, 52)
  line L18 (-128, 52) -> (-132, 52)
  line L19 (-132, 52) -> (-132, 68)
  line L20 (97, -68) -> (113, -68)
  line L21 (113, -68) -> (113, -72)
  line L22 (113, -72) -> (97, -72)
  line L23 (97, -72) -> (97, -68)
  circle A0 centre (-92.7583, -134.6621) radius 2.15
  circle A1 centre (92.7583, -134.6621) radius 2.15
  circle A2 centre (-31, 138) radius 2.15
  circle A3 centre (15, 52) radius 2.15
  circle A4 centre (-31, 52) radius 2.15
  circle A5 centre (15, 138) radius 2.15
  circle A6 centre (78.9019, -142.6621) radius 2.15
  circle A7 centre (-78.9019, -142.6621) radius 2.15
  circle A8 centre (-109, 65) radius 1.6
  circle A9 centre (-105, 142.5) radius 1.6
  circle A10 centre (105, -63) radius 1.6
  circle A11 centre (-123, 60) radius 1.6
  circle A12 centre (-105, -63) radius 1.6
  circle A13 centre (123, 60) radius 1.6
  circle A14 centre (105, 142.5) radius 1.6
  circle A15 centre (-72, 65) radius 1.6
  line L24 (87, 175.4) -> (72, 175.4)
  arc A16 (72, 178.6) -> (72, 175.4) centre (72, 177) ccw
  line L25 (72, 178.6) -> (87, 178.6)
  arc A17 (87, 175.4) -> (87, 178.6) centre (87, 177) ccw
  line L26 (-20, 119) -> (-20, 107)
  line L27 (-20, 107) -> (-28, 107)
  line L28 (-28, 107) -> (-28, 119)
  line L29 (-28, 119) -> (-20, 119)
  line L30 (-131.8869, -67.9327) -> (-141.7167, -74.8156)
  line L31 (-141.7167, -74.8156) -> (-146.3053, -68.2624)
  line L32 (-146.3053, -68.2624) -> (-136.4755, -61.3795)
  line L33 (-136.4755, -61.3795) -> (-131.8869, -67.9327)
  line L34 (-114.185, -114.1349) -> (-118.7736, -107.5817)
  line L35 (-118.7736, -107.5817) -> (-108.9438, -100.6988)
  line L36 (-108.9438, -100.6988) -> (-104.3552, -107.252)
  line L37 (-104.3552, -107.252) -> (-114.185, -114.1349)
  line L38 (28, 107) -> (20, 107)
  line L39 (20, 107) -> (20, 119)
  line L40 (20, 119) -> (28, 119)
  line L41 (28, 119) -> (28, 107)
  arc A18 (115.4, 162) -> (118.6, 162) centre (117, 162) ccw
  line L42 (115.4, 162) -> (115.4, 177)
  arc A19 (118.6, 177) -> (115.4, 177) centre (117, 177) ccw
  line L43 (118.6, 177) -> (118.6, 162)
  line L44 (-118.6, 162) -> (-118.6, 177)
  arc A20 (-115.4, 177) -> (-118.6, 177) centre (-117, 177) ccw
  line L45 (-115.4, 177) -> (-115.4, 162)
  arc A21 (-118.6, 162) -> (-115.4, 162) centre (-117, 162) ccw
  line L46 (141.7167, -74.8156) -> (131.8869, -67.9327)
  line L47 (131.8869, -67.9327) -> (136.4755, -61.3795)
  line L48 (136.4755, -61.3795) -> (146.3053, -68.2624)
  line L49 (146.3053, -68.2624) -> (141.7167, -74.8156)
  line L50 (-18.3661, -106.8973) -> (-23.2142, -98.1511)
  line L51 (-23.2142, -98.1511) -> (-17.0919, -94.7574)
  arc A22 (-12.2438, -103.5036) -> (-17.0919, -94.7574) centre (0, -91) ccw
  line L52 (-12.2438, -103.5036) -> (-18.3661, -106.8973)
  line L53 (104.3552, -107.252) -> (108.9438, -100.6988)
  line L54 (108.9438, -100.6988) -> (118.7736, -107.5817)
  line L55 (118.7736, -107.5817) -> (114.185, -114.1349)
  line L56 (114.185, -114.1349) -> (104.3552, -107.252)
  arc A23 (-72, 175.4) -> (-72, 178.6) centre (-72, 177) ccw
  line L57 (-72, 175.4) -> (-87, 175.4)
  arc A24 (-87, 178.6) -> (-87, 175.4) centre (-87, 177) ccw
  line L58 (-87, 178.6) -> (-72, 178.6)
  line L59 (-75, 72) -> (-75, 58)
  arc A25 (-78, 55) -> (-75, 58) centre (-78, 58) ccw
  line L60 (-78, 55) -> (-103, 55)
  arc A26 (-106, 58) -> (-103, 55) centre (-103, 58) ccw
  line L61 (-106, 58) -> (-106, 72)
  arc A27 (-103, 75) -> (-106, 72) centre (-103, 72) ccw
  line L62 (-103, 75) -> (-78, 75)
  arc A28 (-75, 72) -> (-78, 75) centre (-78, 72) ccw
  circle A29 centre (-15, 125) radius 1.6
  circle A30 centre (-53.5096, -122.6814) radius 1.6
  circle A31 centre (-40, -17) radius 1.6
  circle A32 centre (-66, -45.5) radius 1.6
  circle A33 centre (30, 8) radius 1.6
  circle A34 centre (-30, -52) radius 1.6
  circle A35 centre (110, 67) radius 1.6
  circle A36 centre (90, 32) radius 1.6
  circle A37 centre (122.4607, -104.0595) radius 1.6
  circle A38 centre (-122.4607, -104.0595) radius 1.6
  circle A39 centre (77, 49.5) radius 1.6
  circle A40 centre (45, -10) radius 1.6
  circle A41 centre (-80, -40) radius 1.6
  circle A42 centre (60, -40) radius 1.6
  circle A43 centre (104.1506, -130.3942) radius 1.6
  circle A44 centre (-60.8494, -155.3942) radius 1.6
  circle A45 centre (-104.1506, -130.3942) radius 1.6
  circle A46 centre (-31, -163) radius 1.6
  circle A47 centre (25, -106) radius 1.6
  circle A48 centre (-25, -106) radius 1.6
  circle A49 centre (31, -163) radius 1.6
  circle A50 centre (-93.1506, -111.3416) radius 1.6
  circle A51 centre (60.8494, -155.3942) radius 1.6
  circle A52 centre (93.1507, -111.3416) radius 1.6
  circle A53 centre (102, -40) radius 1.6
  circle A54 centre (-122, -40) radius 1.6
  circle A55 centre (77, -10) radius 1.6
  circle A56 centre (45, 49.5) radius 1.6
  circle A57 centre (-139.668, -79.4849) radius 1.6
  circle A58 centre (139.668, -79.4849) radius 1.6
  circle A59 centre (110, 32) radius 1.6
  circle A60 centre (90, 67) radius 1.6
  circle A61 centre (-30, 8) radius 1.6
  circle A62 centre (30, -52) radius 1.6
  circle A63 centre (-40, -45.5) radius 1.6
  circle A64 centre (-66, -17) radius 1.6
  circle A65 centre (53.5096, -122.6814) radius 1.6
  circle A66 centre (15, 125) radius 1.6
  arc A67 (68.2426, 187) -> (66.1213, 186.1213) centre (68.2426, 184) ccw
  line L63 (66.1213, 186.1213) -> (32.8787, 152.8787)
  arc A68 (30.7574, 152) -> (32.8787, 152.8787) centre (30.7574, 155) ccw
  line L64 (30.7574, 152) -> (-30.7574, 152)
  arc A69 (-32.8787, 152.8787) -> (-30.7574, 152) centre (-30.7574, 155) ccw
  line L65 (-32.8787, 152.8787) -> (-66.1213, 186.1213)
  arc A70 (-66.1213, 186.1213) -> (-68.2426, 187) centre (-68.2426, 184) ccw
  line L66 (-68.2426, 187) -> (-121.307, 187)
  arc A71 (-121.307, 187) -> (-123.7177, 185.7857) centre (-121.307, 184) ccw
  line L67 (-123.7177, 185.7857) -> (-168.7454, 125)
  arc A72 (-168.7454, 125) -> (-189.8044, 89.8571) centre (0, 0) ccw
  arc A73 (-189.8044, 89.8571) -> (-189.9662, 87.7108) centre (-187.0929, 88.5734) ccw
  line L68 (-189.9662, 87.7108) -> (-186.7921, 77.1374)
  arc A74 (-186.7921, 77.1374) -> (-183.9188, 75) centre (-183.9188, 78) ccw
  line L69 (-183.9188, 75) -> (-162, 75)
  arc A75 (-159, 72) -> (-162, 75) centre (-162, 72) ccw
  line L70 (-159, 72) -> (-159, -72)
  arc A76 (-162, -75) -> (-159, -72) centre (-162, -72) ccw
  line L71 (-162, -75) -> (-163.331, -75)
  arc A77 (-163.331, -75) -> (-166.0381, -79.2928) centre (-163.331, -78) ccw
  arc A78 (-166.0381, -79.2928) -> (166.0381, -79.2928) centre (0, 0) ccw
  arc A79 (166.0381, -79.2928) -> (163.331, -75) centre (163.331, -78) ccw
  line L72 (163.331, -75) -> (162, -75)
  arc A80 (159, -72) -> (162, -75) centre (162, -72) ccw
  line L73 (159, -72) -> (159, 72)
  arc A81 (162, 75) -> (159, 72) centre (162, 72) ccw
  line L74 (162, 75) -> (183.9188, 75)
  arc A82 (183.9188, 75) -> (186.7921, 77.1374) centre (183.9188, 78) ccw
  line L75 (186.7921, 77.1374) -> (189.9662, 87.7108)
  arc A83 (189.9662, 87.7108) -> (189.8044, 89.8571) centre (187.0929, 88.5734) ccw
  arc A84 (189.8044, 89.8571) -> (168.7454, 125) centre (0, 0) ccw
  line L76 (168.7454, 125) -> (123.7177, 185.7857)
  arc A85 (123.7177, 185.7857) -> (121.307, 187) centre (121.307, 184) ccw
  line L77 (121.307, 187) -> (68.2426, 187)
  circle A86 centre (0, 0) radius 200
  circle A87 centre (0, 210) radius 75
  line L78 (60.2662, 254.6429) -> (160.7099, 119.0476)
  line L79 (0, 0) -> (178.2013, 90.7981)
  line L80 (0, 0) -> (0, 210)
  line L81 (0, 0) -> (-178.2013, 90.7981)
  line L82 (-60.2662, 254.6429) -> (-160.7099, 119.0476)
  point P0 (132.7337, 156.8144)
  point P1 (-132.7337, 156.8144)
  dimension "d206" = 400
  dimension "d207" = 150
  dimension "d210" = 210
  dimension "d211" = 47
  dimension "d212" = 63
  dimension "d213" = 63
  dimension "d214" = 47
  constraint coincident A72.centre A78.centre
  constraint vertical A72.centre A87.centre
  constraint coincident A87 L78.start
  constraint coincident A86 L78.end
  constraint tangent A87 L78
  constraint tangent A86 L78
  constraint coincident L78 P0
  constraint coincident A86 L79.end
  constraint coincident A87.centre L80.end
  constraint coincident A86 L81.end
  constraint coincident A87 L82.start
  constraint coincident A86 L82.end
  constraint tangent A87 L82
  constraint tangent A86 L82
  constraint coincident L82 P1
  measures "d206" diameter of A86
  measures "d207" diameter of A87
  measures "d210" distance of A72.centre A87.centre
  measures "d211" distance of L78.end P0
  measures "d212" angle of L79 L80
  measures "d213" angle of L80 L81
  measures "d214" distance of L82.end P1
hole "穴9" at (-178.2013, 0, 90.7981) at (178.2013, 0, 90.7981) at (132.7337, 0, 156.8144) at (-132.7337, 0, 156.8144) direction (0, 1, 0) diameter 3.2 end through all
hole "穴10" at (-65, 5, 35) at (-117, 5, 35) direction (0, -1, 0) diameter 3.2 depth 35 tip angle 118
hole "穴11" at (-149.05, 5, -15.6) at (-149.05, 5, 15.6) at (149.05, 5, -15.6) at (149.05, 5, 15.6) direction (0, -1, 0) diameter 6 depth 80 tip angle 118
equation "d4 = ( ( 37.5 + 23 ) * 2 ) * 1 mm"
